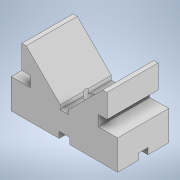
# Autodesk Inventor part: 부품1
Saved by Autodesk Inventor 2022 (Build 260153000, 153)
## iProperties
Created: 2022-08-22
Part Number: 부품1
Material: 일반
Document SubType Name: Modeling
Designer: USER
Density: 1 g/cm^3
Appearance: 기본값
Author: USER
Autodesk Inventor part; units mm, degrees
ref_plane "YZ Plane" through (0, 0, 0) normal (1, 0, 0) x (0, 1, 0)
ref_plane "XZ Plane" through (0, 0, 0) normal (0, 1, 0) x (-1, 0, 0)
ref_plane "XY Plane" through (0, 0, 0) normal (0, 0, 1) x (1, 0, 0)
sketch "스케치1" plane through (0, 0, 0) normal (0, 0, 1) x (1, 0, 0)
  line L0 (50, 0) -> (50, 28)
  line L1 (-50, 28) -> (-50, 0)
  line L2 (32, 28) -> (32, 38)
  line L3 (-32, 38) -> (-32, 28)
  line L4 (-40, 38) -> (-40, 60)
  line L5 (40, 60) -> (40, 38)
  line L6 (-35.94, 60) -> (-3.94, 28)
  line L7 (3.94, 28) -> (35.94, 60)
  line L8 (-40, 60) -> (-35.94, 60)
  line L9 (35.94, 60) -> (40, 60)
  line L10 (3.94, 28) -> (4.06, 28)
  line L11 (4.06, 28) -> (4.06, 24.06)
  line L12 (4.06, 24.06) -> (-3.94, 24.06)
  line L13 (-3.94, 24.06) -> (-3.94, 28)
  line L14 (-32, 28) -> (-3.94, 28)
  line L15 (3.94, 28) -> (32, 28)
  line L16 (50, 28) -> (3.94, 28)
  line L17 (-3.94, 28) -> (-50, 28)
  line L18 (32, 38) -> (13.94, 38)
  line L19 (-13.94, 38) -> (-32, 38)
  line L20 (40, 38) -> (13.94, 38)
  line L21 (-13.94, 38) -> (-40, 38)
  line L22 (4.06, 0) -> (5, 0)
  line L23 (5, 0) -> (5, 5.8283)
  line L24 (5, 5.8283) -> (-5, 5.8283)
  line L25 (-5, 5.8283) -> (-5, 0)
  line L26 (-50, 0) -> (-5, 0)
  line L27 (5, 0) -> (50, 0)
  point P0 (0, 0)
  point P1 (0, 0)
  dimension "d0" = 100
  dimension "d1" = 28
  dimension "d2" = 50
  dimension "d3" = 64
  dimension "d4" = 32
  dimension "d5" = 10
  dimension "d6" = 80
  dimension "d8" = 40
  dimension "d11" = 90
  dimension "d12" = 80
  dimension "d13" = 4.06
  dimension "d14" = 4.06
  dimension "d15" = 8
  dimension "d16" = 10
  dimension "d17" = 5
  constraints: 56 end point, 19 parallel, 8 horizontal, 8 perpendicular, 4 point on line, 1 coincident
  measures "d0" distance of L1.start L0.end
  measures "d1" distance of L0.end L0.start
  measures "d2" distance from line of L1 point (0, 0)
  measures "d3" distance of L3.start L2.end
  measures "d4" distance from line of L3 point (0, 0)
  measures "d5" distance of L2.start L2.end
  measures "d6" distance between parallel lines of L5 L4
  measures "d8" distance from line of point (0, 0) L4
  measures "d11" angle of L7 L6
  measures "d12" distance of L4.end L5.start
  measures "d13" distance of L4.end L6.start
  measures "d14" distance of L7.end L5.start
  measures "d15" distance of L11.end L12.end
  measures "d16" distance of L24.end L23.end
  measures "d17" distance from line of point (0, 0) L25
extrude "돌출1" add sketch "스케치1" along normal mid plane 48
sketch "스케치2" plane through (50, 0, 24) normal (1, 0, 0) x (0, 0, -1)
  line L0 (48, 0) -> (0, 0) projected
  line L1 (48, 5.8283) -> (0, 5.8283) projected
  line L2 (19.5, 0) -> (28.5, 0)
  line L3 (28.5, 0) -> (28.5, 5.8283)
  line L4 (28.5, 5.8283) -> (19.5, 5.8283)
  line L5 (19.5, 5.8283) -> (19.5, 0)
  point P0 (24, 0)
  dimension "d20" = 9
  dimension "d21" = 4.5
  constraints: 8 end point, 2 parallel, 2 point on line, 1 horizontal, 1 perpendicular
  measures "d20" distance of L4.end L3.end
  measures "d21" distance from line of L5 point (24, 0)
extrude "돌출2" cut sketch "스케치2" against normal through all
sketch "스케치3" plane through (-5, 5.8283, 24) normal (0, -1, 0) x (1, 0, 0)
  circle A0 centre (5, -24) radius 4.5
  dimension "d24" = 9
  constraints: 1 centre point, 1 coincident
  measures "d24" diameter of A0
extrude "돌출3" cut sketch "스케치3" against normal through all
